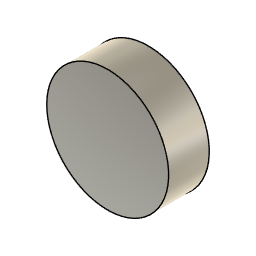
magnet (Autodesk Fusion 360 design; units mm, degrees)
Autodesk Fusion 360 part; units mm, degrees
sketch "Sketch1" plane through (0, 0.5, 0) normal (0, -1, 0) x (1, 0, 0)
  circle A0 centre (11.8655, -35.668) radius 3
  circle A1 centre (11.8655, -35.668) radius 1.5
extrude "Extrude1" add sketch "Sketch1" along normal up to surface (2 mm away) contours A0 | A1
